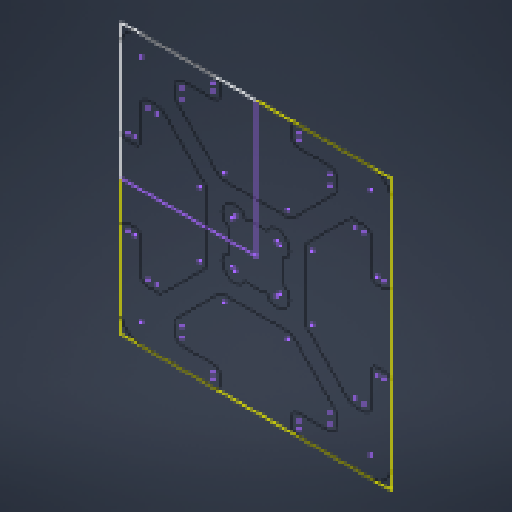
# Autodesk Inventor part: 2020_extrusion
Saved by Autodesk Inventor 2024 (Build 280153000, 153)
## iProperties
Created: 2026-03-28
Part Number: 2020_extrusion
Material: Generic
Document SubType Name: Modeling
Designer: schar
Density: 1 g/cm^3
Appearance: Default
Author: schar
Autodesk Inventor part; units mm, degrees
ref_plane "YZ Plane" through (0, 0, 0) normal (1, 0, 0) x (0, 1, 0)
ref_plane "XZ Plane" through (0, 0, 0) normal (0, 1, 0) x (-1, 0, 0)
sketch "Sketch1" plane through (0, 0, 0) normal (0, 0, 1) x (1, 0, 0)
  line L0 (0, 0) -> (20, 0) projected
  line L1 (20, 0) -> (20, 20) projected
  line L2 (0, 20) -> (20, 20) projected
  line L3 (0, 0) -> (0, 20) projected
  line L4 (0, 20) -> (10, 20)
  line L5 (10, 20) -> (10, 10)
  line L6 (10, 10) -> (0, 10)
  line L7 (0, 10) -> (0, 20)
  arc A0 (10.804, 8.0649) -> (12.1249, 7.6955) centre (11.5684, 8.252) ccw
  line L8 (12.1249, 7.6955) -> (12.3045, 7.8751)
  arc A1 (12.3045, 7.8751) -> (11.9351, 9.196) centre (11.748, 8.4316) ccw
  arc A2 (11.9351, 9.196) -> (11.9351, 10.804) centre (10, 10) ccw
  arc A3 (11.9351, 10.804) -> (12.3045, 12.1249) centre (11.748, 11.5684) ccw
  line L9 (12.3045, 12.1249) -> (12.1249, 12.3045)
  arc A4 (12.1249, 12.3045) -> (10.804, 11.9351) centre (11.5684, 11.748) ccw
  arc A5 (10.804, 11.9351) -> (9.196, 11.9351) centre (10, 10) ccw
  arc A6 (9.196, 11.9351) -> (7.8751, 12.3045) centre (8.4316, 11.748) ccw
  line L10 (7.8751, 12.3045) -> (7.6955, 12.1249)
  arc A7 (7.6955, 12.1249) -> (8.0649, 10.804) centre (8.252, 11.5684) ccw
  arc A8 (8.0649, 10.804) -> (8.0649, 9.196) centre (10, 10) ccw
  arc A9 (8.0649, 9.196) -> (7.6955, 7.8751) centre (8.252, 8.4316) ccw
  line L11 (7.6955, 7.8751) -> (7.8751, 7.6955)
  arc A10 (7.8751, 7.6955) -> (9.196, 8.0649) centre (8.4316, 8.252) ccw
  arc A11 (9.196, 8.0649) -> (10.804, 8.0649) centre (10, 10) ccw
  line L12 (19.008, 12.63) -> (19.492, 12.63)
  arc A12 (18.5, 13.138) -> (19.008, 12.63) centre (19.008, 13.138) ccw
  line L13 (18.5, 15.487) -> (18.5, 13.138)
  arc A13 (18.5, 15.487) -> (17.992, 15.995) centre (17.992, 15.487) ccw
  line L14 (17.2661, 15.995) -> (17.992, 15.995)
  arc A14 (17.2661, 15.995) -> (16.9069, 15.8462) centre (17.2661, 15.487) ccw
  line L15 (13.8038, 12.7431) -> (16.9069, 15.8462)
  arc A15 (13.8038, 12.7431) -> (13.655, 12.3839) centre (14.163, 12.3839) ccw
  line L16 (13.655, 7.6161) -> (13.655, 12.3839)
  arc A16 (13.655, 7.6161) -> (13.8038, 7.2569) centre (14.163, 7.6161) ccw
  line L17 (16.9069, 4.1538) -> (13.8038, 7.2569)
  arc A17 (16.9069, 4.1538) -> (17.2661, 4.005) centre (17.2661, 4.513) ccw
  line L18 (17.992, 4.005) -> (17.2661, 4.005)
  arc A18 (17.992, 4.005) -> (18.5, 4.513) centre (17.992, 4.513) ccw
  line L19 (18.5, 6.862) -> (18.5, 4.513)
  arc A19 (19.008, 7.37) -> (18.5, 6.862) centre (19.008, 6.862) ccw
  line L20 (19.492, 7.37) -> (19.008, 7.37)
  arc A20 (20, 6.862) -> (19.492, 7.37) centre (19.492, 6.862) ccw
  line L21 (20, 1.5) -> (20, 6.862)
  arc A21 (18.5, 0) -> (20, 1.5) centre (18.5, 1.5) ccw
  line L22 (13.138, 0) -> (18.5, 0)
  arc A22 (12.63, 0.508) -> (13.138, 0) centre (13.138, 0.508) ccw
  line L23 (12.63, 0.992) -> (12.63, 0.508)
  arc A23 (13.138, 1.5) -> (12.63, 0.992) centre (13.138, 0.992) ccw
  line L24 (15.487, 1.5) -> (13.138, 1.5)
  arc A24 (15.487, 1.5) -> (15.995, 2.008) centre (15.487, 2.008) ccw
  line L25 (15.995, 2.7339) -> (15.995, 2.008)
  arc A25 (15.995, 2.7339) -> (15.8462, 3.0931) centre (15.487, 2.7339) ccw
  line L26 (12.7431, 6.1962) -> (15.8462, 3.0931)
  arc A26 (12.7431, 6.1962) -> (12.3839, 6.345) centre (12.3839, 5.837) ccw
  line L27 (7.6161, 6.345) -> (12.3839, 6.345)
  arc A27 (7.6161, 6.345) -> (7.2569, 6.1962) centre (7.6161, 5.837) ccw
  line L28 (4.1538, 3.0931) -> (7.2569, 6.1962)
  arc A28 (4.1538, 3.0931) -> (4.005, 2.7339) centre (4.513, 2.7339) ccw
  line L29 (4.005, 2.008) -> (4.005, 2.7339)
  arc A29 (4.005, 2.008) -> (4.513, 1.5) centre (4.513, 2.008) ccw
  line L30 (6.862, 1.5) -> (4.513, 1.5)
  arc A30 (7.37, 0.992) -> (6.862, 1.5) centre (6.862, 0.992) ccw
  line L31 (7.37, 0.508) -> (7.37, 0.992)
  arc A31 (6.862, 0) -> (7.37, 0.508) centre (6.862, 0.508) ccw
  line L32 (1.5, 0) -> (6.862, 0)
  arc A32 (0, 1.5) -> (1.5, 0) centre (1.5, 1.5) ccw
  line L33 (0, 6.862) -> (0, 1.5)
  arc A33 (0.508, 7.37) -> (0, 6.862) centre (0.508, 6.862) ccw
  line L34 (0.992, 7.37) -> (0.508, 7.37)
  arc A34 (1.5, 6.862) -> (0.992, 7.37) centre (0.992, 6.862) ccw
  line L35 (1.5, 4.513) -> (1.5, 6.862)
  arc A35 (1.5, 4.513) -> (2.008, 4.005) centre (2.008, 4.513) ccw
  line L36 (2.7339, 4.005) -> (2.008, 4.005)
  arc A36 (2.7339, 4.005) -> (3.0931, 4.1538) centre (2.7339, 4.513) ccw
  line L37 (6.1962, 7.2569) -> (3.0931, 4.1538)
  arc A37 (6.1962, 7.2569) -> (6.345, 7.6161) centre (5.837, 7.6161) ccw
  line L38 (6.345, 12.3839) -> (6.345, 7.6161)
  arc A38 (6.345, 12.3839) -> (6.1962, 12.7431) centre (5.837, 12.3839) ccw
  line L39 (3.0931, 15.8462) -> (6.1962, 12.7431)
  arc A39 (3.0931, 15.8462) -> (2.7339, 15.995) centre (2.7339, 15.487) ccw
  line L40 (2.008, 15.995) -> (2.7339, 15.995)
  arc A40 (2.008, 15.995) -> (1.5, 15.487) centre (2.008, 15.487) ccw
  line L41 (1.5, 13.138) -> (1.5, 15.487)
  arc A41 (0.992, 12.63) -> (1.5, 13.138) centre (0.992, 13.138) ccw
  line L42 (0.508, 12.63) -> (0.992, 12.63)
  arc A42 (0, 13.138) -> (0.508, 12.63) centre (0.508, 13.138) ccw
  line L43 (0, 18.5) -> (0, 13.138)
  arc A43 (1.5, 20) -> (0, 18.5) centre (1.5, 18.5) ccw
  line L44 (6.862, 20) -> (1.5, 20)
  arc A44 (7.37, 19.492) -> (6.862, 20) centre (6.862, 19.492) ccw
  line L45 (7.37, 19.008) -> (7.37, 19.492)
  arc A45 (6.862, 18.5) -> (7.37, 19.008) centre (6.862, 19.008) ccw
  line L46 (4.513, 18.5) -> (6.862, 18.5)
  arc A46 (4.513, 18.5) -> (4.005, 17.992) centre (4.513, 17.992) ccw
  line L47 (4.005, 17.2661) -> (4.005, 17.992)
  arc A47 (4.005, 17.2661) -> (4.1538, 16.9069) centre (4.513, 17.2661) ccw
  line L48 (7.2569, 13.8038) -> (4.1538, 16.9069)
  arc A48 (7.2569, 13.8038) -> (7.6161, 13.655) centre (7.6161, 14.163) ccw
  line L49 (12.3839, 13.655) -> (7.6161, 13.655)
  arc A49 (12.3839, 13.655) -> (12.7431, 13.8038) centre (12.3839, 14.163) ccw
  line L50 (15.8462, 16.9069) -> (12.7431, 13.8038)
  arc A50 (15.8462, 16.9069) -> (15.995, 17.2661) centre (15.487, 17.2661) ccw
  line L51 (15.995, 17.992) -> (15.995, 17.2661)
  arc A51 (15.995, 17.992) -> (15.487, 18.5) centre (15.487, 17.992) ccw
  line L52 (13.138, 18.5) -> (15.487, 18.5)
  arc A52 (12.63, 19.008) -> (13.138, 18.5) centre (13.138, 19.008) ccw
  line L53 (12.63, 19.492) -> (12.63, 19.008)
  arc A53 (13.138, 20) -> (12.63, 19.492) centre (13.138, 19.492) ccw
  line L54 (18.5, 20) -> (13.138, 20)
  arc A54 (20, 18.5) -> (18.5, 20) centre (18.5, 18.5) ccw
  line L55 (20, 13.138) -> (20, 18.5)
  arc A55 (19.492, 12.63) -> (20, 13.138) centre (19.492, 13.138) ccw
  point P0 (8.0649, 10.804)
  point P1 (7.8751, 12.3045)
  point P2 (9.196, 11.9351)
  point P3 (10.804, 11.9351)
  point P4 (12.3045, 12.1249)
  point P5 (11.9351, 10.804)
  point P6 (11.9351, 9.196)
  point P7 (12.1249, 7.6955)
  point P8 (10.804, 8.0649)
  point P9 (9.196, 8.0649)
  point P10 (7.6955, 7.8751)
  point P11 (8.0649, 9.196)
  point P12 (3.0931, 4.1538)
  point P13 (2.008, 4.005)
  point P14 (1.5, 6.862)
  point P15 (0.508, 7.37)
  point P16 (0, 1.5)
  point P17 (6.862, 0)
  point P18 (7.37, 0.508)
  point P19 (7.37, 0.992)
  point P20 (4.513, 1.5)
  point P21 (4.005, 2.7339)
  point P22 (7.2569, 6.1962)
  point P23 (12.3839, 6.345)
  point P24 (15.8462, 3.0931)
  point P25 (15.995, 2.008)
  point P26 (13.138, 1.5)
  point P27 (12.63, 0.508)
  point P28 (18.5, 0)
  point P29 (20, 6.862)
  point P30 (19.492, 7.37)
  point P31 (19.008, 7.37)
  point P32 (18.5, 4.513)
  point P33 (17.2661, 4.005)
  point P34 (13.8038, 7.2569)
  point P35 (13.655, 12.3839)
  point P36 (16.9069, 15.8462)
  point P37 (17.992, 15.995)
  point P38 (18.5, 13.138)
  point P39 (19.492, 12.63)
  point P40 (20, 18.5)
  point P41 (13.138, 20)
  point P42 (12.63, 19.492)
  point P43 (12.63, 19.008)
  point P44 (15.487, 18.5)
  point P45 (15.995, 17.2661)
  point P46 (12.7431, 13.8038)
  point P47 (4.1538, 16.9069)
  point P48 (4.005, 17.992)
  point P49 (6.862, 18.5)
  point P50 (7.37, 19.492)
  point P51 (1.5, 20)
  point P52 (0, 13.138)
  point P53 (0.508, 12.63)
  point P54 (0.992, 12.63)
  point P55 (1.5, 15.487)
  point P56 (2.7339, 15.995)
  point P57 (6.1962, 12.7431)
  constraints: 112 point on circle, 104 end point, 56 centre point, 2 parallel, 1 horizontal, 1 perpendicular
ref_plane "Work Plane1" through (-70.9931, -4.3, 93.5988) normal (0, 0, -1) x (0, 1, 0)
extrude "Extrusion1" add sketch "Sketch1" along normal up to surface (93.5988 mm away) contours A32 L3 A33 L34 A34 L35 A35 L36 A36 L37 A37 L38 L6 A8 A9 L11 A10 A11 A0 L8 A1 A2 A3 L9 A4 A5 L5 L49 A49 L50 A50 L51 A51 L52 A52 L53 A53 L2 A54 L1 A55 L12 A12 L13 A13 L14 A14 L15 A15 L16 A16 L17 A17 L18 A18 L19 A19 L20 A20 A21 L0 A22 L23 A23 L24 A24 L25 A25 L26 A26 L27 A27 L28 A28 L29 A29 L30 A30 L31 A31 | L3 A43 L2 A44 L45 A45 L46 A46 L47 A47 L48 A48 L49 L5 A5 A6 L10 A7 A8 L6 L38 A38 L39 A39 L40 A40 L41 A41 L42 A42
body "Solid1"
